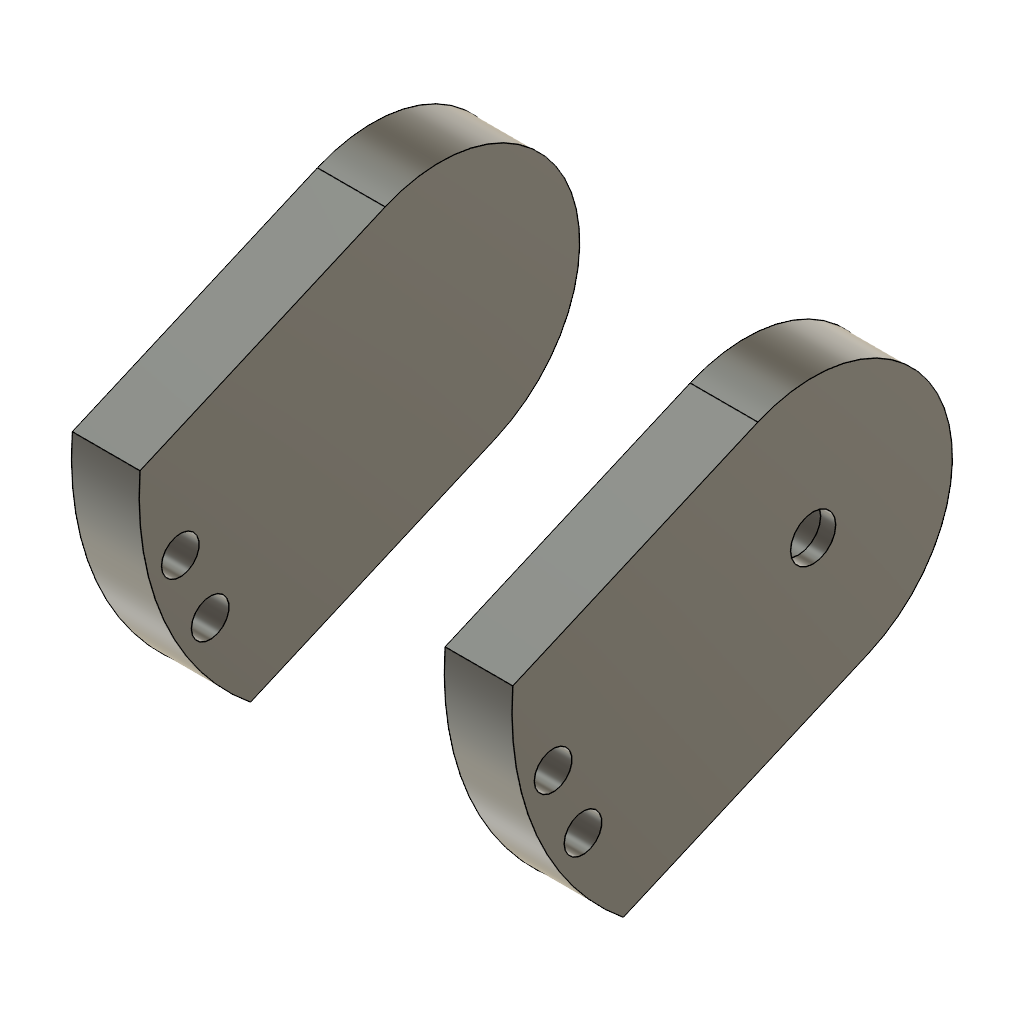
weapon-arms (Autodesk Fusion 360 design; units mm, degrees)
Autodesk Fusion 360 part; units mm, degrees
sketch "arm-weapon" plane through (0, 0, 0) normal (1, 0, 0) x (0, 1, 0)
  circle A0 centre (0, 0) radius 40
  line L0 (-39.8938, 2.9124) -> (-7.3393, 16.9819)
  line L1 (-25.2153, -31.0514) -> (7.3393, -16.9819)
  arc A1 (7.3393, -16.9819) -> (-7.3393, 16.9819) centre (0, 0) ccw
  line L2 (-7.3393, 16.9819) -> (0, 0)
  circle A2 centre (0, 0) radius 14.5
  line L3 (-8.416, -11.8077) -> (-14.3667, 1.9614)
  line L4 (-14.3667, 1.9614) -> (-28.1358, -3.9893)
  line L5 (-28.1358, -3.9893) -> (-22.1851, -17.7585)
  line L6 (-22.1851, -17.7585) -> (-8.416, -11.8077)
  line L7 (-11.3913, -4.9231) -> (0, 0)
  line L8 (-39.8938, 2.9124) -> (-25.2153, -31.0514)
  circle A3 centre (-34.5381, -9.4798) radius 2.5
  circle A4 centre (-30.571, -18.6592) radius 2.5
  point P0 (-32.5546, -14.0695)
  dimension "d1" = 80
  dimension "d2" = 29
  dimension "d3" = 4
  dimension "d9" = 15
  dimension "d11" = 15
  dimension "d12" = 5
  dimension "d13" = 5
  dimension "d14" = 5
  dimension "d15" = 5
  constraint coincident A0.centre A1.centre
  constraint coincident A0 L0.start
  constraint coincident A0 L1.start
  constraint parallel L0 L1
  constraint coincident L1.end A1.start
  constraint collinear L0.end L1.end A0.centre
  constraint perpendicular L0 L2
  constraint concentric A1 A2
  constraint coincident A2 L3.start
  constraint coincident A2 L3.end
  constraint parallel L3 L5
  constraint parallel L4 L6
  constraint parallel L0 L4
  constraint midpoint L3 L7.start
  constraint parallel L4 L7
  constraint midpoint L8 P0
  constraint coincident L8 A3.centre
  constraint coincident L8 A4.centre
  measures "d1" diameter of A0
  measures "d2" diameter of A2
  measures "d3" distance of A1 A2
  measures "d9" distance of L3.start L5.end
  measures "d11" distance of L4.end L5.end
  measures "d12" diameter of A3
  measures "d13" diameter of A4
  measures "d14" distance of P0 A3.centre
  measures "d15" distance of P0 A4.centre
extrude "Extrude1" add sketch "arm-weapon" along normal blind 2.5 contours A0 L8 A3 A4 | L0 L1 A1 L8 A3 A4 | L2 A2 L3 L7 | L2 A2 L3 L7 | A2 L3 | A2 L4 L5 L6 makes body 1
extrude "Extrude2" add sketch "arm-weapon" against normal blind 6.5 contours A0 L8 A3 A4 | L0 L1 A1 L8 A3 A4 bodies 1
sketch "Sketch2" plane through (0, 0, 0) normal (1, 0, 0) x (0, 1, 0)
  circle A0 centre (0, 0) radius 39.993
  circle A1 centre (0, 0) radius 18.5
  line L0 (-7.3393, 16.9819) -> (-39.8866, 2.9155)
  line L1 (-25.208, -31.0483) -> (7.3393, -16.9819)
  line L2 (-39.8866, 2.9155) -> (-25.208, -31.0483)
  circle A2 centre (-34.5309, -9.4767) radius 2.5
  circle A3 centre (-30.5637, -18.6561) radius 2.5
  circle A4 centre (0, 0) radius 4
  circle A5 centre (0, 0) radius 3
  point P0 (-7.3393, 16.9819)
  point P1 (-32.5473, -14.0664)
  dimension "d16" = 5
  dimension "d17" = 5
  dimension "d18" = 5
  dimension "d19" = 5
  dimension "d20" = 8
  dimension "d21" = 1
  constraint coincident A0.centre A1.centre
  constraint concentric A0 A1
  constraint coincident A1 P0
  constraint coincident P0 L0.start
  constraint coincident A0 L0.end
  constraint tangent A1 L0
  constraint coincident A0 L1.start
  constraint coincident A1 L1.end
  constraint tangent A1 L1
  constraint parallel L0 L1
  constraint midpoint L2 P1
  constraint coincident L2 A2.centre
  constraint coincident L2 A3.centre
  constraint concentric A1 A4
  constraint concentric A1 A5
  measures "d16" diameter of A2
  measures "d17" diameter of A3
  measures "d18" distance of P1 A2.centre
  measures "d19" distance of P1 A3.centre
  measures "d20" diameter of A4
  measures "d21" distance of A4 A5
extrude "Extrude3" add sketch "Sketch2" along normal blind 2 separate body contours A0 L2 A2 A3 | A1 L0 L1 L2 A2 A3 | A1 | A4 makes body 2
extrude "Extrude4" add sketch "Sketch2" against normal blind 7 contours A0 L2 A2 A3 | A1 L0 L1 L2 A2 A3 | A1 bodies 2
move_body "Move1" bodies 2 to x (1, 0, 0) y (0, 1, 0) z (0, 0, 1) at (50, 0, 0)
